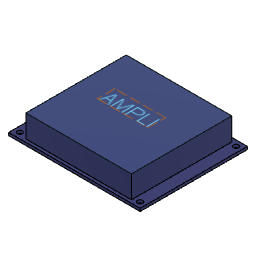
Enceinte bass reflex 12mm v8 (Autodesk Fusion 360 archive; units mm, degrees)
design "Ampli BT 5.0 XH-A353"
Autodesk Fusion 360 part; units mm, degrees
sketch "Esquisse1" plane through (0, 0, 0) normal (0, 1, 0) x (1, 0, 0)
  circle A0 centre (0, 0) radius 1.5
  circle A1 centre (69.5, 0) radius 1.5
  circle A2 centre (0, -55.5) radius 1.5
  circle A3 centre (69.5, -55.5) radius 1.5
  line L0 (-3.25, -58.75) -> (72.75, -58.75)
  line L1 (72.75, -58.75) -> (72.75, 3.25)
  line L2 (72.75, 3.25) -> (-3.25, 3.25)
  line L3 (-3.25, 3.25) -> (-3.25, -58.75)
  point P0 (34.75, -27.75)
  dimension "d1" = 3
  dimension "d2" = 3
  dimension "d3" = 69.5
  dimension "d4" = 3
  dimension "d5" = 55.5
  dimension "d6" = 3
  dimension "d7" = 76
  dimension "d8" = 62
  constraint coincident A0.centre origin
  constraint horizontal L0
  constraint perpendicular L0 L1
  constraint parallel L0 L2
  constraint parallel L1 L3
  measures "d1" diameter of A0
  measures "d2" diameter of A1
  measures "d3" distance of A0.centre A1.centre
  measures "d4" diameter of A2
  measures "d5" distance of A0.centre A2.centre
  measures "d6" diameter of A3
  measures "d7" distance of L1.end L2.end
  measures "d8" distance of L0.end L1.end
extrude "Extrusion1" add sketch "Esquisse1" along normal blind 1.6 makes body 1
sketch "Esquisse2" plane through (0, 1.6, 0) normal (0, 1, 0) x (-1, 0, 0)
  circle A0 centre (0, 55.5) radius 1.5
  circle A1 centre (-69.5, 55.5) radius 1.5
  circle A2 centre (0, 0) radius 1.5
  circle A3 centre (-69.5, 0) radius 1.5
  line L0 (3.25, -3.25) -> (3.25, 58.75)
  line L1 (3.25, 58.75) -> (-72.75, 58.75)
  line L2 (-72.75, 58.75) -> (-72.75, -3.25)
  line L3 (-72.75, -3.25) -> (3.25, -3.25)
  line L4 (-5, -1) -> (-66, -1)
  line L5 (-66, -1) -> (-66, 57)
  line L6 (-66, 57) -> (-5, 57)
  line L7 (-5, 57) -> (-5, -1)
  constraint horizontal L4
  constraint vertical L5
  constraint horizontal L6
  constraint vertical L7
extrude "Extrusion2" add sketch "Esquisse2" along normal blind 13 separate body contours L4 L5 L6 L7 makes body 2
sketch "Esquisse3" plane through (0, 14.6, 0) normal (0, 1, 0) x (-1, 0, 0)
  line L0 (-5, 57) -> (-66, 57)
  line L1 (-66, 57) -> (-66, -1)
  line L2 (-66, -1) -> (-5, -1)
  line L3 (-5, -1) -> (-5, 57)
  line L4 (-18.5635, 29.1796) -> (-47.6894, 29.1796) construction
  line L5 (-47.6894, 29.1796) -> (-47.6894, 19.1796) construction
  line L6 (-47.6894, 19.1796) -> (-18.5635, 19.1796) construction
  line L7 (-18.5635, 19.1796) -> (-18.5635, 29.1796) construction
  constraint perpendicular L4 L5
  constraint parallel L4 L6
  constraint parallel L5 L7

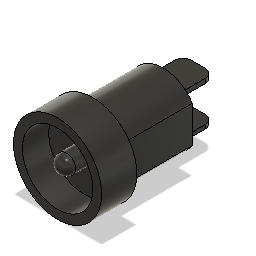
design "Embase alimentation DC"
Autodesk Fusion 360 part; units mm, degrees
sketch "Esquisse1" plane through (0, 0, 0) normal (0, 0, 1) x (1, 0, 0)
  circle A0 centre (0, 0) radius 5
  dimension "d1" = 10
  constraint coincident A0.centre origin
  measures "d1" diameter of A0
extrude "Extrusion1" add sketch "Esquisse1" along normal blind 4 makes body 1
sketch "Esquisse2" plane through (0, 0, 0) normal (0, 0, -1) x (-1, 0, 0)
  circle A0 centre (0, 0) radius 5
  line L0 (-3.3, 2.0785) -> (-3.3, -2.0785)
  line L1 (3.3, -2.0785) -> (3.3, 2.0785)
  line L2 (3.3, 2.8288) -> (-3.3, -2.8288) construction
  line L3 (-2.961, 2.5382) -> (3.3, -2.8288) construction
  arc A1 (-3.3, -2.0785) -> (3.3, -2.0785) centre (0, 0) ccw
  arc A2 (3.3, 2.0785) -> (-3.3, 2.0785) centre (0, 0) ccw
  dimension "d4" = 7.8
  dimension "d5" = 6.6
  constraint coincident A0.centre A1.centre
  constraint parallel L0 L1
  constraint coincident L2 A0.centre
  constraint coincident L3 A0.centre
  constraint concentric A1 A2
  constraint coincident A2 L3.start
  measures "d4" diameter of A1
  measures "d5" distance of L2.end L3.end
extrude "Extrusion2" add sketch "Esquisse2" along normal blind 8 contours L0 L1 A1 A2 bodies 1
sketch "Esquisse3" plane through (0, 0, 4) normal (0, 0, 1) x (1, 0, 0)
  circle A0 centre (0, 0) radius 5
  circle A1 centre (0, 0) radius 4
  constraint coincident A0.centre A1.centre
extrude "Extrusion3" cut sketch "Esquisse3" against normal blind 3 contours A1 bodies 1
sketch "Esquisse4" plane through (0, 0, 1) normal (0, 0, 1) x (1, 0, 0)
  circle A0 centre (0, 0) radius 4
  circle A1 centre (0, 0) radius 1.05
  dimension "d10" = 2.1
  constraint coincident A0.centre A1.centre
  measures "d10" diameter of A1
extrude "Extrusion4" add sketch "Esquisse4" along normal blind 3 contours A1 bodies 1
fillet "Congé1" radius 1 1 edges at (-0.9789, -0.3797, 4) on bodies 1
copy_body "Corps->Comp1" bodies 1 removing the originals makes body 2 in component "Component"
sketch "Esquisse5" plane through (0, 0, -8) normal (0, 0, -1) x (-1, 0, 0)
  arc A0 (3.3, 2.0785) -> (-3.3, 2.0785) centre (0, 0) ccw
  line L0 (-3.3, 2.0785) -> (-3.3, -2.0785)
  arc A1 (-3.3, -2.0785) -> (3.3, -2.0785) centre (0, 0) ccw
  line L1 (3.3, -2.0785) -> (3.3, 2.0785)
  line L2 (1.7624, 1.7418) -> (-1.7624, 1.7418)
  line L3 (-1.7624, 1.7418) -> (-1.7624, 2.2582)
  line L4 (-1.7624, 2.2582) -> (1.7624, 2.2582)
  line L5 (1.7624, 2.2582) -> (1.7624, 1.7418)
  line L6 (1.7624, 1.7418) -> (-1.7624, 2.2582) construction
  line L7 (-1.7624, 1.7418) -> (1.7624, 2.2582) construction
  line L8 (1.7624, -2.2778) -> (-1.7624, -2.2778)
  line L9 (-1.7624, -2.2778) -> (-1.7624, -2.7222)
  line L10 (-1.7624, -2.7222) -> (1.7624, -2.7222)
  line L11 (1.7624, -2.7222) -> (1.7624, -2.2778)
  line L12 (1.7624, -2.2778) -> (-1.7624, -2.7222) construction
  line L13 (-1.7624, -2.2778) -> (1.7624, -2.7222) construction
  point P0 (0, 2)
  point P1 (0, -2.5)
  constraint horizontal L2
  constraint perpendicular L2 L3
  constraint parallel L2 L4
  constraint parallel L3 L5
  constraint coincident L6 P0
  constraint coincident L7 P0
  constraint horizontal L8
  constraint perpendicular L8 L9
  constraint parallel L8 L10
  constraint parallel L9 L11
  constraint coincident L12 P1
  constraint coincident L13 P1
extrude "Extrusion1'" add sketch "Esquisse5" along normal blind 4 contours L2 L3 L4 L5 | L8 L9 L10 L11 bodies 2 in component "Component"
fillet "Congé1'" radius 1 4 edges at (-1.7624, 2, -12) (1.7624, 2, -12) (1.7624, -2.5, -12) (-1.7624, -2.5, -12) on bodies 2 in component "Component"
component "Component" placed x (1, 0, 0) y (0, 1, 0) z (0, 0, 1) at (0, 0, 0)

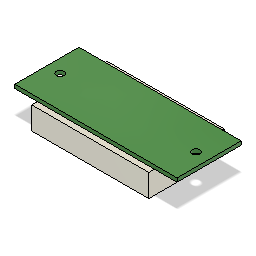
design "Niveau batterie MH-DL 18S"
Autodesk Fusion 360 part; units mm, degrees
sketch "Esquisse1" plane through (0, 0, 0) normal (0, 1, 0) x (1, 0, 0)
  line L0 (15.5, -10) -> (-15.5, -10)
  line L1 (-15.5, -10) -> (-15.5, 10)
  line L2 (-15.5, 10) -> (15.5, 10)
  line L3 (15.5, 10) -> (15.5, -10)
  line L4 (15.5, -10) -> (-15.5, 10) construction
  line L5 (-15.5, -10) -> (15.5, 10) construction
  dimension "d1" = 31
  dimension "d2" = 20
  constraint horizontal L0
  constraint perpendicular L0 L1
  constraint parallel L0 L2
  constraint parallel L1 L3
  constraint coincident L4 origin
  constraint coincident L5 origin
  measures "d1" distance of L1.end L2.end
  measures "d2" distance of L0.end L1.end
extrude "Extrusion1" add sketch "Esquisse1" along normal blind 6 makes body 1
copy_body "Corps->Comp1" bodies 1 removing the originals makes body 2 in component "Segments LED"
sketch "Esquisse1 (2)" plane through (0, 6, 0) normal (0, 1, 0) x (-1, 0, 0) in component "Cirduit imprimé"
  line L0 (-15.5, -10) -> (15.5, -10)
  line L1 (15.5, -10) -> (15.5, 10)
  line L2 (15.5, 10) -> (-15.5, 10)
  line L3 (-15.5, 10) -> (-15.5, -10)
  line L4 (21.5, -8.5) -> (-21.5, -8.5)
  line L5 (-21.5, -8.5) -> (-21.5, 8.5)
  line L6 (-21.5, 8.5) -> (21.5, 8.5)
  line L7 (21.5, 8.5) -> (21.5, -8.5)
  line L8 (21.5, -8.5) -> (-21.5, 8.5) construction
  line L9 (-21.5, -8.5) -> (21.5, 8.5) construction
  dimension "d5" = 43
  constraint horizontal L4
  constraint perpendicular L4 L5
  constraint parallel L4 L6
  constraint parallel L5 L7
  constraint coincident L8 origin
  constraint coincident L9 origin
  measures "d5" distance of L5.end L6.end
extrude "Extrusion1'" add sketch "Esquisse1 (2)" along normal blind 1 separate body contours L3 L4 L5 L6 | L1 L3 L4 L6 | L1 L4 L6 L7 makes body 3 in component "Cirduit imprimé"
sketch "Esquisse2" plane through (0, 7, 0) normal (0, 1, 0) x (-1, 0, 0) in component "Cirduit imprimé"
  line L0 (21.5, 8.5) -> (-21.5, 8.5)
  line L1 (-21.5, 8.5) -> (-21.5, -8.5)
  line L2 (-21.5, -8.5) -> (21.5, -8.5)
  line L3 (21.5, -8.5) -> (21.5, 8.5)
  line L4 (24, 0) -> (-26, 0) construction
  circle A0 centre (-18, 0) radius 1
  circle A1 centre (18, 0) radius 1
  line L5 (0, -10.5) -> (0, 8.5) construction
  dimension "d8" = 2
  dimension "d9" = 2
  dimension "d10" = 36
  dimension "d11" = 18
  constraint horizontal L4
  constraint coincident L4 A0.centre
  constraint coincident L4 A1.centre
  constraint midpoint L0 L5.end
  constraint perpendicular L0 L5
  measures "d8" diameter of A0
  measures "d9" diameter of A1
  measures "d10" distance of A0.centre A1.centre
  measures "d11" distance of origin A1.centre
extrude "Extrusion2" cut sketch "Esquisse2" against normal blind 2 contours A0 | A1 bodies 3 in component "Cirduit imprimé"
sketch "Esquisse1 (3)" plane through (0, 0, 0) normal (0, -1, 0) x (1, 0, 0) in component "Component'"
  line L0 (-15.5, -10) -> (15.5, -10)
  line L1 (15.5, -10) -> (15.5, 10)
  line L2 (15.5, 10) -> (-15.5, 10)
  line L3 (-15.5, 10) -> (-15.5, -10)
  line L4 (-9.5, 3.5) -> (-6.5, 3.5)
  line L5 (-6.5, 3.5) -> (-6.5, -3.5)
  line L6 (-6.5, -3.5) -> (-9.5, -3.5)
  line L7 (-9.5, -3.5) -> (-9.5, 3.5)
  line L8 (-9.5, 3.5) -> (-6.5, -3.5) construction
  line L9 (-6.5, 3.5) -> (-9.5, -3.5) construction
  line L10 (-1.1667, 3.5) -> (-4.1667, -3.5) construction
  line L11 (-1.1667, 3.5) -> (-1.1667, -3.5)
  line L12 (-1.1667, -3.5) -> (-4.1667, -3.5)
  line L13 (-4.1667, 3.5) -> (-1.1667, -3.5) construction
  line L14 (-4.1667, -3.5) -> (-4.1667, 3.5)
  line L15 (-4.1667, 3.5) -> (-1.1667, 3.5)
  line L16 (4.1667, 3.5) -> (1.1667, -3.5) construction
  line L17 (4.1667, 3.5) -> (4.1667, -3.5)
  line L18 (4.1667, -3.5) -> (1.1667, -3.5)
  line L19 (1.1667, 3.5) -> (4.1667, -3.5) construction
  line L20 (1.1667, -3.5) -> (1.1667, 3.5)
  line L21 (1.1667, 3.5) -> (4.1667, 3.5)
  line L22 (9.5, 3.5) -> (6.5, -3.5) construction
  line L23 (9.5, 3.5) -> (9.5, -3.5)
  line L24 (9.5, -3.5) -> (6.5, -3.5)
  line L25 (6.5, 3.5) -> (9.5, -3.5) construction
  line L26 (6.5, -3.5) -> (6.5, 3.5)
  line L27 (6.5, 3.5) -> (9.5, 3.5)
  point P0 (-8, 0)
  point P1 (-2.6667, 0)
  point P2 (2.6667, 0)
  point P3 (8, 0)
  dimension "d14" = 3
  dimension "d15" = 7
  dimension "d18" = 16
  dimension "d19" = 0
  constraint horizontal L4
  constraint perpendicular L4 L5
  constraint parallel L4 L6
  constraint parallel L5 L7
  constraint coincident L8 P0
  constraint coincident L9 P0
  measures "d14" distance of L5.end L6.end
  measures "d15" distance of L4.end L5.end
sketch "Esquisse2 (2)" plane through (0, 0, 0) normal (0, -1, 0) x (1, 0, 0) in component "Component'"
  line L0 (-11, -4) -> (-11, -2)
  line L1 (-11, -2) -> (-12, -2)
  line L2 (-12, -2) -> (-12, -6)
  line L3 (-12, -6) -> (12, -6)
  line L4 (12, -6) -> (12, -2)
  line L5 (12, -2) -> (13, -2)
  line L6 (13, -2) -> (13, 2)
  line L7 (13, 2) -> (12, 2)
  line L8 (12, 2) -> (12, 6)
  line L9 (12, 6) -> (-12, 6)
  line L10 (-12, 6) -> (-12, 2)
  line L11 (-12, 2) -> (-11, 2)
  line L12 (-11, 2) -> (-11, 5)
  line L13 (-11, 5) -> (11, 5)
  line L14 (11, 5) -> (11, -5)
  line L15 (11, -5) -> (-11, -5)
  line L16 (-11, -5) -> (-11, -4)
  constraint vertical L0
  constraint perpendicular L0 L1
  constraint perpendicular L1 L2
  constraint perpendicular L2 L3
  constraint perpendicular L3 L4
  constraint perpendicular L4 L5
  constraint perpendicular L5 L6
  constraint perpendicular L6 L7
  constraint perpendicular L5 L8
  constraint perpendicular L8 L9
  constraint perpendicular L9 L10
  constraint perpendicular L10 L11
  constraint perpendicular L11 L12
  constraint perpendicular L10 L13
  constraint perpendicular L13 L14
  constraint perpendicular L2 L15
  constraint perpendicular L13 L16
extrude "Extrusion1''" add sketch "Esquisse2 (2)" sketch "Esquisse1 (3)" along normal blind 0.1 of sketch 2 contours L4 L5 L6 L7 | L11 L12 L14 L15 | L17 L18 L20 L21 | L23 L24 L26 L27 bodies 2 in component "Segments LED"
component "Segments LED" placed x (1, 0, 0) y (0, 1, 0) z (0, 0, 1) at (0, 0, 0)
component "Cirduit imprimé" placed x (1, 0, 0) y (0, 1, 0) z (0, 0, 1) at (0, 0, 0)
component "Component'" placed x (1, 0, 0) y (0, 1, 0) z (0, 0, 1) at (0, 0, 0)

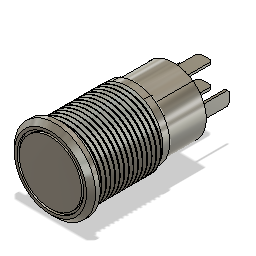
design "Interrupteur 16mm"
Autodesk Fusion 360 part; units mm, degrees
sketch "Esquisse1" plane through (0, 0, 0) normal (0, 0, 1) x (1, 0, 0)
  circle A0 centre (0, 0) radius 8
  dimension "d1" = 16
  constraint coincident A0.centre origin
  measures "d1" diameter of A0
extrude "Extrusion1" add sketch "Esquisse1" along normal blind 15 makes body 1
thread "Filetage1" "ISO Metric profile 16.0 M16x1 6g" major diameter 15.884 minor diameter 14.741 pitch 1 angle 60 modelled right hand crest width 0.1429 on face at (7.9602, -0.7965, 10) crest through (7.942, 0, -0.25) on bodies 1
sketch "Esquisse2" plane through (0, 0, 15) normal (0, 0, 1) x (1, 0, 0)
  spline S0 degree 3 poles (-3.4471, 7.1549) (-4.3561, 6.6775) (-5.1637, 6.0282) (-6.4739, 4.4655) (-6.9677, 3.5705) (-7.578, 1.654) (-7.6936, 0.6526) (-7.5328, -1.3242) (-7.2633, -2.281) (-6.524, -3.7345) (-6.1578, -4.2703) (-5.3004, -5.2291) (-4.8139, -5.6491) (-4.2793, -6.001) knots 0 0 0 0 0.308029 0.308029 0.611955 0.611955 0.911778 0.911778 1.207495 1.207495 1.401599 1.401599 1.593872 1.593872 1.593872 1.593872
  arc A0 (-4.2793, -6.001) -> (4.2793, -6.001) centre (0, 0) ccw
  spline S1 degree 3 poles (4.2793, -6.001) (5.0861, -5.47) (5.7807, -4.7855) (6.8785, -3.1785) (7.2667, -2.2686) (7.678, -0.3379) (7.692, 0.6654) (7.3345, 2.6352) (6.9614, 3.5818) (6.0534, 5.0017) (5.6158, 5.5223) (4.6136, 6.4425) (4.0521, 6.8371) (3.4471, 7.1549) knots 0 0 0 0 0.28978 0.28978 0.58366 0.58366 0.881638 0.881638 1.183715 1.183715 1.386635 1.386635 1.591382 1.591382 1.591382 1.591382
  arc A1 (3.4471, 7.1549) -> (-3.4471, 7.1549) centre (0, 0) ccw
  circle A2 centre (0, 0) radius 8.9
  dimension "d4" = 17.8
  constraint concentric A0 A2
  measures "d4" diameter of A2
extrude "Extrusion2" add sketch "Esquisse2" along normal blind 2 contours S0 A0 S1 A1 | A2 bodies 1
chamfer "Chanfrein1" distance 1 angle 45 1 edges at (-8.2977, -3.2184, 17) measured on face at (2.0127, -1.7373, 17) on bodies 1
sketch "Esquisse3" plane through (0, 0, 0) normal (0, 0, -1) x (-1, 0, 0)
  spline S0 degree 3 poles (4.2793, -6.001) (5.0861, -5.47) (5.7807, -4.7855) (6.8785, -3.1785) (7.2667, -2.2686) (7.678, -0.3379) (7.692, 0.6654) (7.3345, 2.6352) (6.9614, 3.5818) (6.0534, 5.0017) (5.6158, 5.5223) (4.6136, 6.4425) (4.0521, 6.8371) (3.4471, 7.1549) knots 0 0 0 0 0.28978 0.28978 0.58366 0.58366 0.881638 0.881638 1.183715 1.183715 1.386635 1.386635 1.591382 1.591382 1.591382 1.591382
  arc A0 (3.4471, 7.1549) -> (-3.4471, 7.1549) centre (0, 0) ccw
  spline S1 degree 3 poles (-3.4471, 7.1549) (-4.3561, 6.6775) (-5.1637, 6.0282) (-6.4739, 4.4655) (-6.9677, 3.5705) (-7.578, 1.654) (-7.6936, 0.6526) (-7.5328, -1.3242) (-7.2633, -2.281) (-6.524, -3.7345) (-6.1578, -4.2703) (-5.3004, -5.2291) (-4.8139, -5.6491) (-4.2793, -6.001) knots 0 0 0 0 0.308029 0.308029 0.611955 0.611955 0.911778 0.911778 1.207495 1.207495 1.401599 1.401599 1.593872 1.593872 1.593872 1.593872
  arc A1 (-4.2793, -6.001) -> (4.2793, -6.001) centre (0, 0) ccw
  circle A2 centre (0, 0) radius 8
  dimension "d9" = 16
  constraint concentric A0 A2
  measures "d9" diameter of A2
extrude "Extrusion3" add sketch "Esquisse3" along normal blind 2 contours S0 A0 S1 A1 bodies 1
fillet "Congé1" radius 0.5 4 edges at (-7.6202, 0.7923, -2) (0, 7.942, -2) (7.6197, 0.8006, -2) (0, -7.3705, -2) on bodies 1
sketch "Esquisse4" plane through (0, 0, -2) normal (0, 0, -1) x (-1, 0, 0)
  spline S0 degree 3 poles (-3.9966, -5.5885) (-3.9992, -5.5868) (-4.0018, -5.5851) (-4.0044, -5.5833) (-4.2516, -5.4207) (-4.4882, -5.242) (-5.4449, -4.4179) (-6.0424, -3.6314) (-6.7755, -2.0859) (-6.9864, -1.3632) (-7.1394, -0.1643) (-7.1528, 0.3026) (-7.1208, 0.7663) (-7.0889, 1.2306) (-7.0115, 1.6917) (-6.6968, 2.8602) (-6.3909, 3.5488) (-5.465, 4.9898) (-4.7779, 5.6982) (-3.7379, 6.4166) (-3.4842, 6.5703) (-3.2222, 6.7082) knots -1.485386 -1.485386 -1.485386 -1.485386 -1.484452 -1.484452 -1.484452 -1.395682 -1.395682 -1.105649 -1.105649 -0.882546 -0.882546 -0.743107 -0.743107 -0.743107 -0.603487 -0.603487 -0.380094 -0.380094 -0.089684 -0.089684 -0.000868 -0.000868 -0.000868 -0.000868
  arc A0 (-3.9966, -5.5885) -> (3.9966, -5.5885) centre (0, 0) ccw
  spline S1 degree 3 poles (3.2222, 6.7082) (3.4878, 6.5683) (3.745, 6.4123) (4.7867, 5.6901) (5.4722, 4.9812) (6.3954, 3.5399) (6.7001, 2.8515) (7.0131, 1.6834) (7.0899, 1.2225) (7.1214, 0.7585) (7.1528, 0.2951) (7.1389, -0.1715) (6.9849, -1.3693) (6.7735, -2.0914) (6.0398, -3.6353) (5.4423, -4.4208) (4.4865, -5.2433) (4.2507, -5.4213) (4.0044, -5.5833) (4.0018, -5.5851) (3.9992, -5.5868) (3.9966, -5.5885) knots -1.483585 -1.483585 -1.483585 -1.483585 -1.393524 -1.393524 -1.10332 -1.10332 -0.880085 -0.880085 -0.740563 -0.740563 -0.740563 -0.601222 -0.601222 -0.378275 -0.378275 -0.088445 -0.088445 0 0 0 0.000935 0.000935 0.000935 0.000935
  arc A1 (3.2222, 6.7082) -> (-3.2222, 6.7082) centre (0, 0) ccw
  circle A2 centre (0, 0) radius 7.3973
  constraint concentric A0 A2
extrude "Extrusion4" add sketch "Esquisse4" along normal blind 8 contours S0 A0 S1 A2 picked at (-0.1669, -1.2655) bodies 1
sketch "Esquisse5" plane through (0, 0, -10) normal (0, 0, -1) x (-1, 0, 0)
  arc A0 (-3.9966, -5.5885) -> (3.9966, -5.5885) centre (0, 0) ccw
  spline S0 degree 3 poles (3.9966, -5.5885) (3.9992, -5.5868) (4.0018, -5.5851) (4.0044, -5.5833) (4.2507, -5.4213) (4.4865, -5.2433) (5.4423, -4.4208) (6.0398, -3.6353) (6.7735, -2.0914) (6.9849, -1.3693) (7.1389, -0.1715) (7.1528, 0.2951) (7.1214, 0.7585) (7.0899, 1.2225) (7.0131, 1.6834) (6.7001, 2.8515) (6.3954, 3.5399) (5.5267, 4.896) (4.9282, 5.5407) (4.2374, 6.0633) knots -0.000935 -0.000935 -0.000935 -0.000935 0 0 0 0.088445 0.088445 0.378275 0.378275 0.601222 0.601222 0.740563 0.740563 0.740563 0.880085 0.880085 1.10332 1.10332 1.363182 1.363182 1.363182 1.363182
  arc A1 (4.2374, 6.0633) -> (-4.2374, 6.0633) centre (0, 0) ccw
  spline S1 degree 3 poles (-4.2374, 6.0633) (-4.9255, 5.5428) (-5.522, 4.9012) (-6.3909, 3.5488) (-6.6968, 2.8602) (-7.0115, 1.6917) (-7.0889, 1.2306) (-7.1208, 0.7663) (-7.1528, 0.3026) (-7.1394, -0.1643) (-6.9864, -1.3632) (-6.7755, -2.0859) (-6.0424, -3.6314) (-5.4449, -4.4179) (-4.4882, -5.242) (-4.2516, -5.4207) (-4.0044, -5.5833) (-4.0018, -5.5851) (-3.9992, -5.5868) (-3.9966, -5.5885) knots 0.12127 0.12127 0.12127 0.12127 0.380094 0.380094 0.603487 0.603487 0.743107 0.743107 0.743107 0.882546 0.882546 1.105649 1.105649 1.395682 1.395682 1.484452 1.484452 1.484452 1.485386 1.485386 1.485386 1.485386
  line L0 (1.5, -5) -> (-1.5, -5) construction
  line L1 (-1.5, -5) -> (-1.5, 5) construction
  line L2 (-1.5, 5) -> (1.5, 5) construction
  line L3 (1.5, 5) -> (1.5, -5) construction
  line L4 (1.5, -5) -> (-1.5, 5) construction
  line L5 (-1.5, -5) -> (1.5, 5) construction
  line L6 (-1.5, 5) -> (1.5, 5)
  line L7 (1.5, 5) -> (1.5, 4.5)
  line L8 (1.5, 4.5) -> (-1.5, 4.5)
  line L9 (-1.5, 4.5) -> (-1.5, 5)
  line L10 (-1.5, -5) -> (1.5, -5)
  line L11 (1.5, -5) -> (1.5, -4.5)
  line L12 (1.5, -4.5) -> (-1.5, -4.5)
  line L13 (-1.5, -4.5) -> (-1.5, -5)
  line L14 (-1.5, 0.2551) -> (1.5, 0.2551)
  line L15 (1.5, 0.2551) -> (1.5, -0.3)
  line L16 (1.5, -0.3) -> (-1.5, -0.3)
  line L17 (-1.5, -0.3) -> (-1.5, 0.2551)
  line L18 (4.75, 1.5) -> (5.25, 1.5)
  line L19 (5.25, 1.5) -> (5.25, -1.5)
  line L20 (5.25, -1.5) -> (4.75, -1.5)
  line L21 (4.75, -1.5) -> (4.75, 1.5)
  line L22 (4.75, 1.5) -> (5.25, -1.5) construction
  line L23 (5.25, 1.5) -> (4.75, -1.5) construction
  line L24 (-5.25, 1.5) -> (-4.75, 1.5)
  line L25 (-4.75, 1.5) -> (-4.75, -1.5)
  line L26 (-4.75, -1.5) -> (-5.25, -1.5)
  line L27 (-5.25, -1.5) -> (-5.25, 1.5)
  line L28 (-5.25, 1.5) -> (-4.75, -1.5) construction
  line L29 (-4.75, 1.5) -> (-5.25, -1.5) construction
  point P0 (5, 0)
  point P1 (-5, 0)
  dimension "d15" = 0.5
  dimension "d16" = 3
  dimension "d17" = 0.5
  dimension "d18" = 3
  constraint horizontal L0
  constraint perpendicular L0 L1
  constraint parallel L0 L2
  constraint parallel L1 L3
  constraint coincident L4 A0.centre
  constraint coincident L5 A0.centre
  constraint coincident A0.centre A1.centre
  constraint horizontal L6
  constraint vertical L7
  constraint horizontal L8
  constraint vertical L9
  constraint coincident L3 L7.end
  constraint horizontal L10
  constraint vertical L11
  constraint horizontal L12
  constraint vertical L13
  constraint coincident L3 L11.end
  constraint horizontal L14
  constraint vertical L15
  constraint horizontal L16
  constraint vertical L17
  constraint coincident L3 L15.end
  constraint horizontal L18
  constraint perpendicular L18 L19
  constraint parallel L18 L20
  constraint parallel L19 L21
  constraint coincident L22 P0
  constraint coincident L23 P0
  constraint horizontal L24
  constraint perpendicular L24 L25
  constraint parallel L24 L26
  constraint parallel L25 L27
  constraint coincident L28 P1
  constraint coincident L29 P1
  measures "d15" distance of L19.end L20.end
  measures "d16" distance of L18.end L19.end
  measures "d17" distance of L25.end L26.end
  measures "d18" distance of L24.end L25.end
extrude "Extrusion5" add sketch "Esquisse5" along normal blind 7 contours L6 L7 L8 L9 | L10 L11 L12 L13 | L14 L15 L16 L17 | L18 L19 L20 L21 | L24 L25 L26 L27 bodies 1
chamfer "Chanfrein2" distance 0.5 angle 45 10 edges at (-1.5, 4.75, -17) (1.5, 4.75, -17) (-5, -1.5, -17) (-5, 1.5, -17) (-1.5, -0.0224, -17) (1.5, -0.0224, -17) (5, 1.5, -17) (5, -1.5, -17) (1.5, -4.75, -17) (-1.5, -4.75, -17) on bodies 1
sketch "Esquisse6" plane through (0, 0, 17) normal (0, 0, 1) x (1, 0, 0)
  circle A0 centre (0, 0) radius 7.9
  circle A1 centre (0, 0) radius 7.2893
  circle A2 centre (0, 0) radius 6.8312
  constraint concentric A0 A1
  constraint concentric A0 A2
extrude "Extrusion6" cut sketch "Esquisse6" against normal blind 0.5 contours A1 bodies 1
copy_body "Corps->Comp1" bodies 1 removing the originals makes body 2 in component "INTERRUPTEUR 16mm"
component "INTERRUPTEUR 16mm" placed x (1, 0, 0) y (0, 1, 0) z (0, 0, 1) at (0, 0, 0)

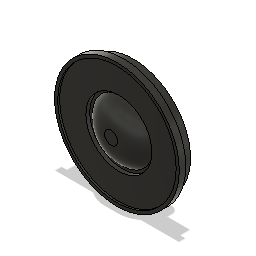
design "Tweeter 20W 6Ohm"
Autodesk Fusion 360 part; units mm, degrees
sketch "Esquisse1" plane through (0, 0, 0) normal (0, 0, 1) x (1, 0, 0)
  circle A0 centre (0, 0) radius 32.1
  dimension "d1" = 64.2
  constraint coincident A0.centre origin
  measures "d1" diameter of A0
extrude "Extrusion1" add sketch "Esquisse1" against normal blind 3.4 makes body 1
sketch "Esquisse2" plane through (0, 0, 0) normal (0, 0, 1) x (1, 0, 0)
  circle A0 centre (0, 0) radius 32.1
  circle A1 centre (0, 0) radius 30.5
  dimension "d4" = 61
  constraint coincident A0.centre A1.centre
  measures "d4" diameter of A1
extrude "Extrusion2" cut sketch "Esquisse2" against normal blind 1 contours A1 bodies 1
sketch "Esquisse3" plane through (0, 0, -1) normal (0, 0, 1) x (1, 0, 0)
  circle A0 centre (0, 0) radius 30.5
  circle A1 centre (0, 0) radius 17
  dimension "d7" = 34
  constraint coincident A0.centre A1.centre
  measures "d7" diameter of A1
extrude "Extrusion3" cut sketch "Esquisse3" against normal blind 2 contours A1 bodies 1
sketch "Esquisse4" plane through (0, 0, -3) normal (0, 0, 1) x (1, 0, 0)
  circle A0 centre (0, 0) radius 17
  circle A1 centre (0, 0) radius 15.6205
  constraint coincident A0.centre A1.centre
extrude "Extrusion4" add sketch "Esquisse4" along normal blind 6 contours A1 bodies 1
fillet "Congé1" radius 15.5 1 edges at (-14.5634, -5.6486, 3) on bodies 1
sketch "Esquisse5" plane through (0, 0, -3.4) normal (0, 0, -1) x (-1, 0, 0)
  circle A0 centre (0, 0) radius 32.1
  circle A1 centre (0, 0) radius 29.5
  circle A2 centre (0, 0) radius 28.5
  dimension "d14" = 59
  dimension "d15" = 57
  constraint coincident A0.centre A1.centre
  measures "d14" diameter of A1
  measures "d15" diameter of A2
extrude "Extrusion5" add sketch "Esquisse5" along normal blind 5 contours A1 bodies 1
sketch "Esquisse6" plane through (0, 0, -3.4) normal (0, 0, -1) x (-1, 0, 0)
  circle A0 centre (0, 0) radius 28.5
  circle A1 centre (0, 0) radius 20.95
  circle A2 centre (0, 0) radius 18
  circle A3 centre (0, 0) radius 20.2485
  circle A4 centre (0, 0) radius 19
  dimension "d18" = 41.9
  dimension "d19" = 36
  constraint coincident A0.centre A1.centre
  constraint concentric A1 A2
  constraint concentric A1 A3
  measures "d18" diameter of A1
  measures "d19" diameter of A2
extrude "Extrusion6" add sketch "Esquisse6" along normal blind 5 contours A1 | A4 bodies 1
extrude "Extrusion7" add 1 faces at (-1.9574, 4.5573, -3.4) along direction (0, 0, -1) blind 11 on bodies 1 bodies 1
fillet "Congé2" radius 4 1 edges at (16.7819, -6.5091, -14.4) on bodies 1
copy_body "Corps->Comp1" bodies 1 removing the originals makes body 2 in component "Component"
component "Component" placed x (1, 0, 0) y (0, 1, 0) z (0, 0, 1) at (0, 0, 0)

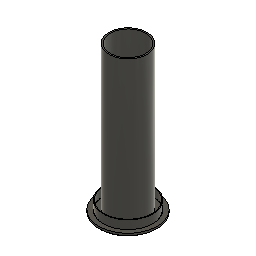
design "Tube bass reflex 26x96"
Autodesk Fusion 360 part; units mm, degrees
sketch "Esquisse1" plane through (0, 0, 0) normal (0, 1, 0) x (1, 0, 0)
  circle A0 centre (0, 0) radius 20.61
  dimension "d1" = 41.22
  constraint coincident A0.centre origin
  measures "d1" diameter of A0
extrude "Extrusion1" add sketch "Esquisse1" along normal blind 1.92 makes body 1
sketch "Esquisse2" plane through (0, 1.92, 0) normal (0, 1, 0) x (-1, 0, 0)
  circle A0 centre (0, 0) radius 20.61
  circle A1 centre (0, 0) radius 17.45
  circle A2 centre (0, 0) radius 16.95
  dimension "d4" = 34.9
  dimension "d5" = 33.9
  constraint coincident A0.centre A1.centre
  constraint concentric A1 A2
  measures "d4" diameter of A1
  measures "d5" diameter of A2
extrude "Extrusion2" add sketch "Esquisse2" along normal blind 6 contours A1 bodies 1
sketch "Esquisse3" plane through (0, 1.92, 0) normal (0, 1, 0) x (-1, 0, 0)
  circle A0 centre (0, 0) radius 16.95
  circle A1 centre (0, 0) radius 13.5
  circle A2 centre (0, 0) radius 12.5
  dimension "d8" = 27
  dimension "d9" = 25
  constraint coincident A0.centre A1.centre
  constraint concentric A1 A2
  measures "d8" diameter of A1
  measures "d9" diameter of A2
extrude "Extrusion3" add sketch "Esquisse3" along normal blind 102 contours A1 bodies 1
extrude "Extrusion4" cut 1 faces at (2.0833, 1.92, 2.3664) along direction (0, -1, 0) blind 10 on bodies 1 bodies 1
fillet "Congé1" radius 4.5 1 edges at (11.6541, 0, -4.5202) on bodies 1
fillet "Congé2" radius 0.5 1 edges at (-19.2153, 0, 7.4529) on bodies 1
copy_body "Corps->Comp1" bodies 1 removing the originals makes body 2 in component "Component"
component "Component" placed x (1, 0, 0) y (0, 1, 0) z (0, 0, 1) at (0, 0, 0)
